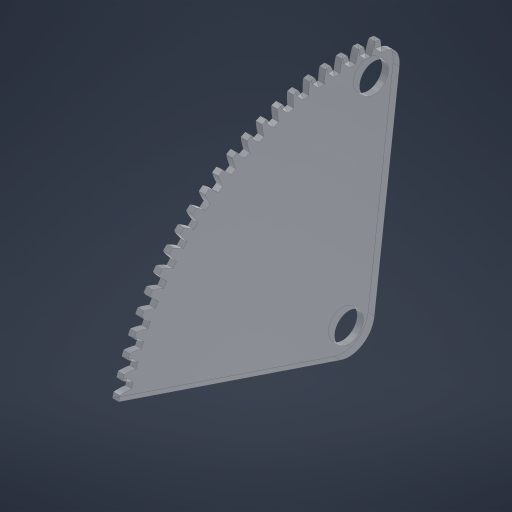
# Autodesk Inventor part: CORL_002_FanPlate
Saved by Autodesk Inventor 2024.2 (Build 282272000, 272)
## iProperties
Created: 2024-08-01
Part Number: CORL_002_FanPlate
Material: Polycarbonate, Clear
Document SubType Name: Modeling
Designer: Bryan
Mass: 353.269 g
Surface Area: 1017.45 cm^2
Volume: 294.391 cm^3
Density: 1.2 g/cm^3
Appearance: Polycarbonate - Clear
Author: Bryan
Autodesk Inventor part; units mm, degrees
ref_plane "YZ Plane" through (0, 0, 0) normal (1, 0, 0) x (0, 1, 0)
ref_plane "XZ Plane" through (0, 0, 0) normal (0, 1, 0) x (-1, 0, 0)
ref_plane "XY Plane" through (0, 0, 0) normal (0, 0, 1) x (1, 0, 0)
sketch "Sketch1" plane through (0, 0, 0) normal (1, 0, 0) x (0, 1, 0)
  circle A0 centre (0, 0) radius 228.6 construction
  circle A1 centre (0, 0) radius 233.68
  circle A2 centre (0, 0) radius 222.25
  line L0 (0, 0) -> (228.6, 0) construction
  line L1 (228.6, 0) -> (214.269, 55.4137) construction
  line L2 (214.269, 55.4137) -> (0, 0) construction
  arc A3 (221.3151, -1.2272) -> (214.269, 55.4137) centre (0, 0) ccw construction
  arc A4 (214.269, 55.4137) -> (209.1377, 72.4107) centre (0, 0) ccw construction
  line L3 (0, 0) -> (222.2162, -3.8788) construction
  line L4 (209.1377, 72.4107) -> (233.6749, 1.542) construction
  spline S0 degree 2 poles (233.6749, 1.542) (228.6917, -0.39) (221.3151, -1.2272) knots 0 0 0 1 1 1
  spline S1 degree 2 poles (233.4787, -9.6962) (228.566, -7.5914) (221.2232, -6.4974) knots 0 0 0 1 1 1
  spline S2 degree 2 poles (232.9981, 17.8386) (228.1618, 15.5636) (220.8616, 14.214) knots 0 0 0 1 1 1
  spline S3 degree 2 poles (233.5864, 6.614) (228.5388, 8.371) (221.1375, 8.9502) knots 0 0 0 1 1 1
  spline S4 degree 2 poles (231.1862, 34.0483) (226.5204, 31.4415) (219.3321, 29.5859) knots 0 0 0 1 1 1
  spline S5 degree 2 poles (232.556, 22.8921) (227.3981, 24.2927) (219.9745, 24.3542) knots 0 0 0 1 1 1
  spline S6 degree 2 poles (228.2479, 50.0921) (223.7753, 47.1662) (216.734, 44.8137) knots 0 0 0 1 1 1
  spline S7 degree 2 poles (230.3926, 39.0586) (225.1496, 40.096) (217.7398, 39.6395) knots 0 0 0 1 1 1
  spline S8 degree 2 poles (224.1977, 65.8918) (219.9401, 62.6611) (213.08, 59.8231) knots 0 0 0 1 1 1
  spline S9 degree 2 poles (227.1068, 55.0348) (221.8042, 55.704) (214.4443, 54.7317) knots 0 0 0 1 1 1
  spline S10 degree 2 poles (219.0552, 81.3706) (215.0333, 77.8507) (208.3879, 74.5411) knots 0 0 0 1 1 1
  spline S11 degree 2 poles (222.7146, 70.7429) (217.3782, 71.0406) (210.104, 69.5573) knots 0 0 0 1 1 1
  spline S12 degree 2 poles (212.8454, 96.4529) (209.0789, 92.661) (202.6806, 88.8959) knots 0 0 0 1 1 1
  spline S13 degree 2 poles (217.2373, 86.1064) (211.8932, 86.0311) (204.7401, 84.0439) knots 0 0 0 1 1 1
  spline S14 degree 2 poles (205.5988, 111.0653) (202.1059, 107.0199) (195.9858, 102.8176) knots 0 0 0 1 1 1
  spline S15 degree 2 poles (210.7016, 101.0504) (205.3758, 100.6024) (198.3788, 98.1211) knots 0 0 0 1 1 1
  spline S16 degree 2 poles (197.3504, 125.1366) (194.1483, 120.8574) (188.3362, 116.2385) knots 0 0 0 1 1 1
  spline S17 degree 2 poles (203.1394, 115.502) (197.8578, 114.6836) (191.051, 111.7203) knots 0 0 0 1 1 1
  spline S18 degree 2 poles (188.1406, 138.5982) (185.2447, 134.1061) (179.769, 129.093) knots 0 0 0 1 1 1
  spline S19 degree 2 poles (194.5876, 129.3909) (189.3759, 128.2061) (182.7923, 124.7752) knots 0 0 0 1 1 1
  spline S20 degree 2 poles (178.0142, 151.3846) (175.4387, 146.7014) (170.326, 141.3186) knots 0 0 0 1 1 1
  spline S21 degree 2 poles (185.0877, 142.6495) (179.9714, 141.104) (173.6432, 137.2222) knots 0 0 0 1 1 1
  spline S22 degree 2 poles (167.0205, 163.4335) (164.778, 158.582) (160.0533, 152.8557) knots 0 0 0 1 1 1
  spline S23 degree 2 poles (174.6861, 155.2131) (169.6901, 153.3145) (163.6481, 149.0007) knots 0 0 0 1 1 1
  spline S24 degree 2 poles (155.2131, 174.6861) (153.3145, 169.6901) (149.0007, 163.6481) knots 0 0 0 1 1 1
  spline S25 degree 2 poles (163.4335, 167.0205) (158.582, 164.778) (152.8557, 160.0533) knots 0 0 0 1 1 1
  spline S26 degree 2 poles (142.6495, 185.0877) (141.104, 179.9714) (137.2222, 173.6432) knots 0 0 0 1 1 1
  spline S27 degree 2 poles (151.3846, 178.0142) (146.7014, 175.4387) (141.3186, 170.326) knots 0 0 0 1 1 1
  spline S28 degree 2 poles (129.3909, 194.5876) (128.2061, 189.3759) (124.7752, 182.7923) knots 0 0 0 1 1 1
  spline S29 degree 2 poles (138.5982, 188.1406) (134.1061, 185.2447) (129.093, 179.769) knots 0 0 0 1 1 1
  spline S30 degree 2 poles (115.502, 203.1394) (114.6836, 197.8578) (111.7203, 191.051) knots 0 0 0 1 1 1
  spline S31 degree 2 poles (125.1366, 197.3504) (120.8574, 194.1483) (116.2385, 188.3362) knots 0 0 0 1 1 1
  spline S32 degree 2 poles (101.0504, 210.7016) (100.6024, 205.3758) (98.1211, 198.3788) knots 0 0 0 1 1 1
  spline S33 degree 2 poles (111.0653, 205.5988) (107.0199, 202.1059) (102.8176, 195.9858) knots 0 0 0 1 1 1
  spline S34 degree 2 poles (86.1064, 217.2373) (86.0311, 211.8932) (84.0439, 204.7401) knots 0 0 0 1 1 1
  spline S35 degree 2 poles (96.4529, 212.8454) (92.661, 209.0789) (88.8959, 202.6806) knots 0 0 0 1 1 1
  spline S36 degree 2 poles (70.7429, 222.7146) (71.0406, 217.3782) (69.5573, 210.104) knots 0 0 0 1 1 1
  spline S37 degree 2 poles (81.3706, 219.0552) (77.8507, 215.0333) (74.5411, 208.3879) knots 0 0 0 1 1 1
  spline S38 degree 2 poles (55.0348, 227.1068) (55.704, 221.8042) (54.7317, 214.4443) knots 0 0 0 1 1 1
  spline S39 degree 2 poles (65.8918, 224.1977) (62.6611, 219.9401) (59.8231, 213.08) knots 0 0 0 1 1 1
  spline S40 degree 2 poles (39.0586, 230.3926) (40.096, 225.1496) (39.6395, 217.7398) knots 0 0 0 1 1 1
  spline S41 degree 2 poles (50.0921, 228.2479) (47.1662, 223.7753) (44.8137, 216.734) knots 0 0 0 1 1 1
  spline S42 degree 2 poles (22.8921, 232.556) (24.2927, 227.3981) (24.3542, 219.9745) knots 0 0 0 1 1 1
  spline S43 degree 2 poles (34.0483, 231.1862) (31.4415, 226.5204) (29.5859, 219.3321) knots 0 0 0 1 1 1
  spline S44 degree 2 poles (6.614, 233.5864) (8.371, 228.5388) (8.9502, 221.1375) knots 0 0 0 1 1 1
  spline S45 degree 2 poles (17.8386, 232.9981) (15.5636, 228.1618) (14.214, 220.8616) knots 0 0 0 1 1 1
  spline S46 degree 2 poles (-9.6962, 233.4787) (-7.5914, 228.566) (-6.4974, 221.2232) knots 0 0 0 1 1 1
  spline S47 degree 2 poles (1.542, 233.6749) (-0.39, 228.6917) (-1.2272, 221.3151) knots 0 0 0 1 1 1
  spline S48 degree 2 poles (-25.9593, 232.2336) (-23.5169, 227.4797) (-21.9133, 220.231) knots 0 0 0 1 1 1
  spline S49 degree 2 poles (-14.7621, 233.2133) (-16.3418, 228.1074) (-16.6623, 220.6904) knots 0 0 0 1 1 1
  spline S50 degree 2 poles (-42.0958, 229.8571) (-39.3278, 225.2851) (-37.2224, 218.166) knots 0 0 0 1 1 1
  spline S51 degree 2 poles (-30.9942, 231.6154) (-32.214, 226.4118) (-32.0163, 218.9905) knots 0 0 0 1 1 1
  spline S52 degree 2 poles (-58.0273, 226.3607) (-54.9471, 221.9929) (-52.3503, 215.038) knots 0 0 0 1 1 1
  spline S53 degree 2 poles (-47.0754, 228.8892) (-47.9292, 223.6132) (-47.2144, 216.2237) knots 0 0 0 1 1 1
  spline S54 degree 2 poles (-73.6761, 221.7615) (-70.2987, 217.6193) (-67.223, 210.8624) knots 0 0 0 1 1 1
  spline S55 degree 2 poles (-62.9272, 225.0478) (-63.4109, 219.7251) (-62.1824, 212.4035) knots 0 0 0 1 1 1
  spline S56 degree 2 poles (-88.9659, 216.0819) (-85.3078, 212.1854) (-81.7683, 205.6595) knots 0 0 0 1 1 1
  spline S57 degree 2 poles (-78.4725, 220.11) (-78.5837, 214.7665) (-76.8474, 207.5485) knots 0 0 0 1 1 1
  spline S58 degree 2 poles (-103.8223, 209.3496) (-99.9013, 205.7177) (-95.9152, 199.4547) knots 0 0 0 1 1 1
  spline S59 degree 2 poles (-93.6354, 214.0999) (-93.3736, 208.7616) (-91.1381, 201.6823) knots 0 0 0 1 1 1
  spline S60 degree 2 poles (-118.1729, 201.5974) (-114.0081, 198.2478) (-109.5948, 192.2781) knots 0 0 0 1 1 1
  spline S61 degree 2 poles (-108.3422, 207.0466) (-107.7086, 201.7397) (-104.9847, 194.8336) knots 0 0 0 1 1 1
  spline S62 degree 2 poles (-131.9478, 192.863) (-127.5594, 189.8121) (-122.7405, 184.1648) knots 0 0 0 1 1 1
  spline S63 degree 2 poles (-122.5211, 198.9847) (-121.5189, 193.7349) (-118.3199, 187.0356) knots 0 0 0 1 1 1
  spline S64 degree 2 poles (-145.0798, 183.189) (-140.4893, 180.4517) (-135.2882, 175.1542) knots 0 0 0 1 1 1
  spline S65 degree 2 poles (-136.1031, 189.9534) (-134.7372, 184.7862) (-131.0786, 178.3264) knots 0 0 0 1 1 1
  spline S66 degree 2 poles (-157.505, 172.6225) (-152.7348, 170.212) (-147.1768, 165.2903) knots 0 0 0 1 1 1
  spline S67 degree 2 poles (-149.0221, 179.9966) (-147.299, 174.9373) (-143.1987, 168.7484) knots 0 0 0 1 1 1
  spline S68 degree 2 poles (-169.1629, 161.215) (-164.2361, 159.1432) (-158.3483, 154.6212) knots 0 0 0 1 1 1
  spline S69 degree 2 poles (-161.215, 169.1629) (-159.1432, 164.2361) (-154.6212, 158.3483) knots 0 0 0 1 1 1
  spline S70 degree 2 poles (-179.9966, 149.0221) (-174.9373, 147.299) (-168.7484, 143.1987) knots 0 0 0 1 1 1
  spline S71 degree 2 poles (-172.6225, 157.505) (-170.212, 152.7348) (-165.2903, 147.1768) knots 0 0 0 1 1 1
  spline S72 degree 2 poles (-189.9534, 136.1031) (-184.7862, 134.7372) (-178.3264, 131.0786) knots 0 0 0 1 1 1
  spline S73 degree 2 poles (-183.189, 145.0798) (-180.4517, 140.4893) (-175.1542, 135.2882) knots 0 0 0 1 1 1
  spline S74 degree 2 poles (-198.9847, 122.5211) (-193.7349, 121.5189) (-187.0356, 118.3199) knots 0 0 0 1 1 1
  spline S75 degree 2 poles (-192.863, 131.9478) (-189.8121, 127.5594) (-184.1648, 122.7405) knots 0 0 0 1 1 1
  spline S76 degree 2 poles (-207.0466, 108.3422) (-201.7397, 107.7086) (-194.8336, 104.9847) knots 0 0 0 1 1 1
  spline S77 degree 2 poles (-201.5974, 118.1729) (-198.2478, 114.0081) (-192.2781, 109.5948) knots 0 0 0 1 1 1
  spline S78 degree 2 poles (-214.0999, 93.6354) (-208.7616, 93.3736) (-201.6823, 91.1381) knots 0 0 0 1 1 1
  spline S79 degree 2 poles (-209.3496, 103.8223) (-205.7177, 99.9013) (-199.4547, 95.9152) knots 0 0 0 1 1 1
  spline S80 degree 2 poles (-220.11, 78.4725) (-214.7665, 78.5837) (-207.5485, 76.8474) knots 0 0 0 1 1 1
  spline S81 degree 2 poles (-216.0819, 88.9659) (-212.1854, 85.3078) (-205.6595, 81.7683) knots 0 0 0 1 1 1
  spline S82 degree 2 poles (-225.0478, 62.9272) (-219.7251, 63.4109) (-212.4035, 62.1824) knots 0 0 0 1 1 1
  spline S83 degree 2 poles (-221.7615, 73.6761) (-217.6193, 70.2987) (-210.8624, 67.223) knots 0 0 0 1 1 1
  spline S84 degree 2 poles (-228.8892, 47.0754) (-223.6132, 47.9292) (-216.2237, 47.2144) knots 0 0 0 1 1 1
  spline S85 degree 2 poles (-226.3607, 58.0273) (-221.9929, 54.9471) (-215.038, 52.3503) knots 0 0 0 1 1 1
  spline S86 degree 2 poles (-231.6154, 30.9942) (-226.4118, 32.214) (-218.9905, 32.0163) knots 0 0 0 1 1 1
  spline S87 degree 2 poles (-229.8571, 42.0958) (-225.2851, 39.3278) (-218.166, 37.2224) knots 0 0 0 1 1 1
  spline S88 degree 2 poles (-233.2133, 14.7621) (-228.1074, 16.3418) (-220.6904, 16.6623) knots 0 0 0 1 1 1
  spline S89 degree 2 poles (-232.2336, 25.9593) (-227.4797, 23.5169) (-220.231, 21.9133) knots 0 0 0 1 1 1
  spline S90 degree 2 poles (-233.6749, -1.542) (-228.6917, 0.39) (-221.3151, 1.2272) knots 0 0 0 1 1 1
  spline S91 degree 2 poles (-233.4787, 9.6962) (-228.566, 7.5914) (-221.2232, 6.4974) knots 0 0 0 1 1 1
  spline S92 degree 2 poles (-232.9981, -17.8386) (-228.1618, -15.5636) (-220.8616, -14.214) knots 0 0 0 1 1 1
  spline S93 degree 2 poles (-233.5864, -6.614) (-228.5388, -8.371) (-221.1375, -8.9502) knots 0 0 0 1 1 1
  spline S94 degree 2 poles (-231.1862, -34.0483) (-226.5204, -31.4415) (-219.3321, -29.5859) knots 0 0 0 1 1 1
  spline S95 degree 2 poles (-232.556, -22.8921) (-227.3981, -24.2927) (-219.9745, -24.3542) knots 0 0 0 1 1 1
  spline S96 degree 2 poles (-228.2479, -50.0921) (-223.7753, -47.1662) (-216.734, -44.8137) knots 0 0 0 1 1 1
  spline S97 degree 2 poles (-230.3926, -39.0586) (-225.1496, -40.096) (-217.7398, -39.6395) knots 0 0 0 1 1 1
  spline S98 degree 2 poles (-224.1977, -65.8918) (-219.9401, -62.6611) (-213.08, -59.8231) knots 0 0 0 1 1 1
  spline S99 degree 2 poles (-227.1068, -55.0348) (-221.8042, -55.704) (-214.4443, -54.7317) knots 0 0 0 1 1 1
  spline S100 degree 2 poles (-219.0552, -81.3706) (-215.0333, -77.8507) (-208.3879, -74.5411) knots 0 0 0 1 1 1
  spline S101 degree 2 poles (-222.7146, -70.7429) (-217.3782, -71.0406) (-210.104, -69.5573) knots 0 0 0 1 1 1
  spline S102 degree 2 poles (-212.8454, -96.4529) (-209.0789, -92.661) (-202.6806, -88.8959) knots 0 0 0 1 1 1
  spline S103 degree 2 poles (-217.2373, -86.1064) (-211.8932, -86.0311) (-204.7401, -84.0439) knots 0 0 0 1 1 1
  spline S104 degree 2 poles (-205.5988, -111.0653) (-202.1059, -107.0199) (-195.9858, -102.8176) knots 0 0 0 1 1 1
  spline S105 degree 2 poles (-210.7016, -101.0504) (-205.3758, -100.6024) (-198.3788, -98.1211) knots 0 0 0 1 1 1
  spline S106 degree 2 poles (-197.3504, -125.1366) (-194.1483, -120.8574) (-188.3362, -116.2385) knots 0 0 0 1 1 1
  spline S107 degree 2 poles (-203.1394, -115.502) (-197.8578, -114.6836) (-191.051, -111.7203) knots 0 0 0 1 1 1
  spline S108 degree 2 poles (-188.1406, -138.5982) (-185.2447, -134.1061) (-179.769, -129.093) knots 0 0 0 1 1 1
  spline S109 degree 2 poles (-194.5876, -129.3909) (-189.3759, -128.2061) (-182.7923, -124.7752) knots 0 0 0 1 1 1
  spline S110 degree 2 poles (-178.0142, -151.3846) (-175.4387, -146.7014) (-170.326, -141.3186) knots 0 0 0 1 1 1
  spline S111 degree 2 poles (-185.0877, -142.6495) (-179.9714, -141.104) (-173.6432, -137.2222) knots 0 0 0 1 1 1
  spline S112 degree 2 poles (-167.0205, -163.4335) (-164.778, -158.582) (-160.0533, -152.8557) knots 0 0 0 1 1 1
  spline S113 degree 2 poles (-174.6861, -155.2131) (-169.6901, -153.3145) (-163.6481, -149.0007) knots 0 0 0 1 1 1
  spline S114 degree 2 poles (-155.2131, -174.6861) (-153.3145, -169.6901) (-149.0007, -163.6481) knots 0 0 0 1 1 1
  spline S115 degree 2 poles (-163.4335, -167.0205) (-158.582, -164.778) (-152.8557, -160.0533) knots 0 0 0 1 1 1
  spline S116 degree 2 poles (-142.6495, -185.0877) (-141.104, -179.9714) (-137.2222, -173.6432) knots 0 0 0 1 1 1
  spline S117 degree 2 poles (-151.3846, -178.0142) (-146.7014, -175.4387) (-141.3186, -170.326) knots 0 0 0 1 1 1
  spline S118 degree 2 poles (-129.3909, -194.5876) (-128.2061, -189.3759) (-124.7752, -182.7923) knots 0 0 0 1 1 1
  spline S119 degree 2 poles (-138.5982, -188.1406) (-134.1061, -185.2447) (-129.093, -179.769) knots 0 0 0 1 1 1
  spline S120 degree 2 poles (-115.502, -203.1394) (-114.6836, -197.8578) (-111.7203, -191.051) knots 0 0 0 1 1 1
  spline S121 degree 2 poles (-125.1366, -197.3504) (-120.8574, -194.1483) (-116.2385, -188.3362) knots 0 0 0 1 1 1
  spline S122 degree 2 poles (-101.0504, -210.7016) (-100.6024, -205.3758) (-98.1211, -198.3788) knots 0 0 0 1 1 1
  spline S123 degree 2 poles (-111.0653, -205.5988) (-107.0199, -202.1059) (-102.8176, -195.9858) knots 0 0 0 1 1 1
  spline S124 degree 2 poles (-86.1064, -217.2373) (-86.0311, -211.8932) (-84.0439, -204.7401) knots 0 0 0 1 1 1
  spline S125 degree 2 poles (-96.4529, -212.8454) (-92.661, -209.0789) (-88.8959, -202.6806) knots 0 0 0 1 1 1
  spline S126 degree 2 poles (-70.7429, -222.7146) (-71.0406, -217.3782) (-69.5573, -210.104) knots 0 0 0 1 1 1
  spline S127 degree 2 poles (-81.3706, -219.0552) (-77.8507, -215.0333) (-74.5411, -208.3879) knots 0 0 0 1 1 1
  spline S128 degree 2 poles (-55.0348, -227.1068) (-55.704, -221.8042) (-54.7317, -214.4443) knots 0 0 0 1 1 1
  spline S129 degree 2 poles (-65.8918, -224.1977) (-62.6611, -219.9401) (-59.8231, -213.08) knots 0 0 0 1 1 1
  spline S130 degree 2 poles (-39.0586, -230.3926) (-40.096, -225.1496) (-39.6395, -217.7398) knots 0 0 0 1 1 1
  spline S131 degree 2 poles (-50.0921, -228.2479) (-47.1662, -223.7753) (-44.8137, -216.734) knots 0 0 0 1 1 1
  spline S132 degree 2 poles (-22.8921, -232.556) (-24.2927, -227.3981) (-24.3542, -219.9745) knots 0 0 0 1 1 1
  spline S133 degree 2 poles (-34.0483, -231.1862) (-31.4415, -226.5204) (-29.5859, -219.3321) knots 0 0 0 1 1 1
  spline S134 degree 2 poles (-6.614, -233.5864) (-8.371, -228.5388) (-8.9502, -221.1375) knots 0 0 0 1 1 1
  spline S135 degree 2 poles (-17.8386, -232.9981) (-15.5636, -228.1618) (-14.214, -220.8616) knots 0 0 0 1 1 1
  spline S136 degree 2 poles (9.6962, -233.4787) (7.5914, -228.566) (6.4974, -221.2232) knots 0 0 0 1 1 1
  spline S137 degree 2 poles (-1.542, -233.6749) (0.39, -228.6917) (1.2272, -221.3151) knots 0 0 0 1 1 1
  spline S138 degree 2 poles (25.9593, -232.2336) (23.5169, -227.4797) (21.9133, -220.231) knots 0 0 0 1 1 1
  spline S139 degree 2 poles (14.7621, -233.2133) (16.3418, -228.1074) (16.6623, -220.6904) knots 0 0 0 1 1 1
  spline S140 degree 2 poles (42.0958, -229.8571) (39.3278, -225.2851) (37.2224, -218.166) knots 0 0 0 1 1 1
  spline S141 degree 2 poles (30.9942, -231.6154) (32.214, -226.4118) (32.0163, -218.9905) knots 0 0 0 1 1 1
  spline S142 degree 2 poles (58.0273, -226.3607) (54.9471, -221.9929) (52.3503, -215.038) knots 0 0 0 1 1 1
  spline S143 degree 2 poles (47.0754, -228.8892) (47.9292, -223.6132) (47.2144, -216.2237) knots 0 0 0 1 1 1
  spline S144 degree 2 poles (73.6761, -221.7615) (70.2987, -217.6193) (67.223, -210.8624) knots 0 0 0 1 1 1
  spline S145 degree 2 poles (62.9272, -225.0478) (63.4109, -219.7251) (62.1824, -212.4035) knots 0 0 0 1 1 1
  spline S146 degree 2 poles (88.9659, -216.0819) (85.3078, -212.1854) (81.7683, -205.6595) knots 0 0 0 1 1 1
  spline S147 degree 2 poles (78.4725, -220.11) (78.5837, -214.7665) (76.8474, -207.5485) knots 0 0 0 1 1 1
  spline S148 degree 2 poles (103.8223, -209.3496) (99.9013, -205.7177) (95.9152, -199.4547) knots 0 0 0 1 1 1
  spline S149 degree 2 poles (93.6354, -214.0999) (93.3736, -208.7616) (91.1381, -201.6823) knots 0 0 0 1 1 1
  spline S150 degree 2 poles (118.1729, -201.5974) (114.0081, -198.2478) (109.5948, -192.2781) knots 0 0 0 1 1 1
  spline S151 degree 2 poles (108.3422, -207.0466) (107.7086, -201.7397) (104.9847, -194.8336) knots 0 0 0 1 1 1
  spline S152 degree 2 poles (131.9478, -192.863) (127.5594, -189.8121) (122.7405, -184.1648) knots 0 0 0 1 1 1
  spline S153 degree 2 poles (122.5211, -198.9847) (121.5189, -193.7349) (118.3199, -187.0356) knots 0 0 0 1 1 1
  spline S154 degree 2 poles (145.0798, -183.189) (140.4893, -180.4517) (135.2882, -175.1542) knots 0 0 0 1 1 1
  spline S155 degree 2 poles (136.1031, -189.9534) (134.7372, -184.7862) (131.0786, -178.3264) knots 0 0 0 1 1 1
  spline S156 degree 2 poles (157.505, -172.6225) (152.7348, -170.212) (147.1768, -165.2903) knots 0 0 0 1 1 1
  spline S157 degree 2 poles (149.0221, -179.9966) (147.299, -174.9373) (143.1987, -168.7484) knots 0 0 0 1 1 1
  spline S158 degree 2 poles (169.1629, -161.215) (164.2361, -159.1432) (158.3483, -154.6212) knots 0 0 0 1 1 1
  spline S159 degree 2 poles (161.215, -169.1629) (159.1432, -164.2361) (154.6212, -158.3483) knots 0 0 0 1 1 1
  spline S160 degree 2 poles (179.9966, -149.0221) (174.9373, -147.299) (168.7484, -143.1987) knots 0 0 0 1 1 1
  spline S161 degree 2 poles (172.6225, -157.505) (170.212, -152.7348) (165.2903, -147.1768) knots 0 0 0 1 1 1
  spline S162 degree 2 poles (189.9534, -136.1031) (184.7862, -134.7372) (178.3264, -131.0786) knots 0 0 0 1 1 1
  spline S163 degree 2 poles (183.189, -145.0798) (180.4517, -140.4893) (175.1542, -135.2882) knots 0 0 0 1 1 1
  spline S164 degree 2 poles (198.9847, -122.5211) (193.7349, -121.5189) (187.0356, -118.3199) knots 0 0 0 1 1 1
  spline S165 degree 2 poles (192.863, -131.9478) (189.8121, -127.5594) (184.1648, -122.7405) knots 0 0 0 1 1 1
  spline S166 degree 2 poles (207.0466, -108.3422) (201.7397, -107.7086) (194.8336, -104.9847) knots 0 0 0 1 1 1
  spline S167 degree 2 poles (201.5974, -118.1729) (198.2478, -114.0081) (192.2781, -109.5948) knots 0 0 0 1 1 1
  spline S168 degree 2 poles (214.0999, -93.6354) (208.7616, -93.3736) (201.6823, -91.1381) knots 0 0 0 1 1 1
  spline S169 degree 2 poles (209.3496, -103.8223) (205.7177, -99.9013) (199.4547, -95.9152) knots 0 0 0 1 1 1
  spline S170 degree 2 poles (220.11, -78.4725) (214.7665, -78.5837) (207.5485, -76.8474) knots 0 0 0 1 1 1
  spline S171 degree 2 poles (216.0819, -88.9659) (212.1854, -85.3078) (205.6595, -81.7683) knots 0 0 0 1 1 1
  spline S172 degree 2 poles (225.0478, -62.9272) (219.7251, -63.4109) (212.4035, -62.1824) knots 0 0 0 1 1 1
  spline S173 degree 2 poles (221.7615, -73.6761) (217.6193, -70.2987) (210.8624, -67.223) knots 0 0 0 1 1 1
  spline S174 degree 2 poles (228.8892, -47.0754) (223.6132, -47.9292) (216.2237, -47.2144) knots 0 0 0 1 1 1
  spline S175 degree 2 poles (226.3607, -58.0273) (221.9929, -54.9471) (215.038, -52.3503) knots 0 0 0 1 1 1
  spline S176 degree 2 poles (231.6154, -30.9942) (226.4118, -32.214) (218.9905, -32.0163) knots 0 0 0 1 1 1
  spline S177 degree 2 poles (229.8571, -42.0958) (225.2851, -39.3278) (218.166, -37.2224) knots 0 0 0 1 1 1
  spline S178 degree 2 poles (233.2133, -14.7621) (228.1074, -16.3418) (220.6904, -16.6623) knots 0 0 0 1 1 1
  spline S179 degree 2 poles (232.2336, -25.9593) (227.4797, -23.5169) (220.231, -21.9133) knots 0 0 0 1 1 1
  point P0 (228.4607, -7.978)
  point P1 (228.0431, 15.9463)
  point P2 (228.4607, 7.978)
  point P3 (226.3753, 31.815)
  point P4 (227.3477, 23.8952)
  point P5 (223.6045, 47.5286)
  point P6 (225.1271, 39.696)
  point P7 (219.7444, 63.0107)
  point P8 (221.8096, 55.3033)
  point P9 (214.8137, 78.1858)
  point P10 (217.4115, 70.6413)
  point P11 (208.8365, 92.98)
  point P12 (211.9542, 85.6351)
  point P13 (201.8418, 107.3212)
  point P14 (205.4643, 100.2116)
  point P15 (193.8638, 121.1395)
  point P16 (197.9734, 114.3)
  point P17 (184.9413, 134.3677)
  point P18 (189.518, 127.8315)
  point P19 (175.1178, 146.9412)
  point P20 (180.1393, 140.7402)
  point P21 (164.4411, 158.7989)
  point P22 (169.8829, 152.9633)
  point P23 (152.9633, 169.8829)
  point P24 (158.7989, 164.4411)
  point P25 (140.7402, 180.1393)
  point P26 (146.9412, 175.1178)
  point P27 (127.8315, 189.518)
  point P28 (134.3677, 184.9413)
  point P29 (114.3, 197.9734)
  point P30 (121.1395, 193.8638)
  point P31 (100.2116, 205.4643)
  point P32 (107.3212, 201.8418)
  point P33 (85.6351, 211.9542)
  point P34 (92.98, 208.8365)
  point P35 (70.6413, 217.4115)
  point P36 (78.1858, 214.8137)
  point P37 (55.3033, 221.8096)
  point P38 (63.0107, 219.7444)
  point P39 (39.696, 225.1271)
  point P40 (47.5286, 223.6045)
  point P41 (23.8952, 227.3477)
  point P42 (31.815, 226.3753)
  point P43 (7.978, 228.4607)
  point P44 (15.9463, 228.0431)
  point P45 (-7.978, 228.4607)
  point P46 (0, 228.6)
  point P47 (-23.8952, 227.3477)
  point P48 (-15.9463, 228.0431)
  point P49 (-39.696, 225.1271)
  point P50 (-31.815, 226.3753)
  point P51 (-55.3033, 221.8096)
  point P52 (-47.5286, 223.6045)
  point P53 (-70.6413, 217.4115)
  point P54 (-63.0107, 219.7444)
  point P55 (-85.6351, 211.9542)
  point P56 (-78.1858, 214.8137)
  point P57 (-100.2116, 205.4643)
  point P58 (-92.98, 208.8365)
  point P59 (-114.3, 197.9734)
  point P60 (-107.3212, 201.8418)
  point P61 (-127.8315, 189.518)
  point P62 (-121.1395, 193.8638)
  point P63 (-140.7402, 180.1393)
  point P64 (-134.3677, 184.9413)
  point P65 (-152.9633, 169.8829)
  point P66 (-146.9412, 175.1178)
  point P67 (-164.4411, 158.7989)
  point P68 (-158.7989, 164.4411)
  point P69 (-175.1178, 146.9412)
  point P70 (-169.8829, 152.9633)
  point P71 (-184.9413, 134.3677)
  point P72 (-180.1393, 140.7402)
  point P73 (-193.8638, 121.1395)
  point P74 (-189.518, 127.8315)
  point P75 (-201.8418, 107.3212)
  point P76 (-197.9734, 114.3)
  point P77 (-208.8365, 92.98)
  point P78 (-205.4643, 100.2116)
  point P79 (-214.8137, 78.1858)
  point P80 (-211.9542, 85.6351)
  point P81 (-219.7444, 63.0107)
  point P82 (-217.4115, 70.6413)
  point P83 (-223.6045, 47.5286)
  point P84 (-221.8096, 55.3033)
  point P85 (-226.3753, 31.815)
  point P86 (-225.1271, 39.696)
  point P87 (-228.0431, 15.9463)
  point P88 (-227.3477, 23.8952)
  point P89 (-228.6, 0)
  point P90 (-228.4607, 7.978)
  point P91 (-228.0431, -15.9463)
  point P92 (-228.4607, -7.978)
  point P93 (-226.3753, -31.815)
  point P94 (-227.3477, -23.8952)
  point P95 (-223.6045, -47.5286)
  point P96 (-225.1271, -39.696)
  point P97 (-219.7444, -63.0107)
  point P98 (-221.8096, -55.3033)
  point P99 (-214.8137, -78.1858)
  point P100 (-217.4115, -70.6413)
  point P101 (-208.8365, -92.98)
  point P102 (-211.9542, -85.6351)
  point P103 (-201.8418, -107.3212)
  point P104 (-205.4643, -100.2116)
  point P105 (-193.8638, -121.1395)
  point P106 (-197.9734, -114.3)
  point P107 (-184.9413, -134.3677)
  point P108 (-189.518, -127.8315)
  point P109 (-175.1178, -146.9412)
  point P110 (-180.1393, -140.7402)
  point P111 (-164.4411, -158.7989)
  point P112 (-169.8829, -152.9633)
  point P113 (-152.9633, -169.8829)
  point P114 (-158.7989, -164.4411)
  point P115 (-140.7402, -180.1393)
  point P116 (-146.9412, -175.1178)
  point P117 (-127.8315, -189.518)
  point P118 (-134.3677, -184.9413)
  point P119 (-114.3, -197.9734)
  point P120 (-121.1395, -193.8638)
  point P121 (-100.2116, -205.4643)
  point P122 (-107.3212, -201.8418)
  point P123 (-85.6351, -211.9542)
  point P124 (-92.98, -208.8365)
  point P125 (-70.6413, -217.4115)
  point P126 (-78.1858, -214.8137)
  point P127 (-55.3033, -221.8096)
  point P128 (-63.0107, -219.7444)
  point P129 (-39.696, -225.1271)
  point P130 (-47.5286, -223.6045)
  point P131 (-23.8952, -227.3477)
  point P132 (-31.815, -226.3753)
  point P133 (-7.978, -228.4607)
  point P134 (-15.9463, -228.0431)
  point P135 (7.978, -228.4607)
  point P136 (0, -228.6)
  point P137 (23.8952, -227.3477)
  point P138 (15.9463, -228.0431)
  point P139 (39.696, -225.1271)
  point P140 (31.815, -226.3753)
  point P141 (55.3033, -221.8096)
  point P142 (47.5286, -223.6045)
  point P143 (70.6413, -217.4115)
  point P144 (63.0107, -219.7444)
  point P145 (85.6351, -211.9542)
  point P146 (78.1858, -214.8137)
  point P147 (100.2116, -205.4643)
  point P148 (92.98, -208.8365)
  point P149 (114.3, -197.9734)
  point P150 (107.3212, -201.8418)
  point P151 (127.8315, -189.518)
  point P152 (121.1395, -193.8638)
  point P153 (140.7402, -180.1393)
  point P154 (134.3677, -184.9413)
  point P155 (152.9633, -169.8829)
  point P156 (146.9412, -175.1178)
  point P157 (164.4411, -158.7989)
  point P158 (158.7989, -164.4411)
  point P159 (175.1178, -146.9412)
  point P160 (169.8829, -152.9633)
  point P161 (184.9413, -134.3677)
  point P162 (180.1393, -140.7402)
  point P163 (193.8638, -121.1395)
  point P164 (189.518, -127.8315)
  point P165 (201.8418, -107.3212)
  point P166 (197.9734, -114.3)
  point P167 (208.8365, -92.98)
  point P168 (205.4643, -100.2116)
  point P169 (214.8137, -78.1858)
  point P170 (211.9542, -85.6351)
  point P171 (219.7444, -63.0107)
  point P172 (217.4115, -70.6413)
  point P173 (223.6045, -47.5286)
  point P174 (221.8096, -55.3033)
  point P175 (226.3753, -31.815)
  point P176 (225.1271, -39.696)
  point P177 (228.0431, -15.9463)
  point P178 (227.3477, -23.8952)
  point P179 (-110.1573, 193.0296)
  point P180 (-118.1729, 201.5974)
  point P181 (229.8571, -42.0958)
  point P182 (219.0645, -37.4939)
  point P183 (219.929, -32.0358)
  point P184 (231.6154, -30.9942)
  point P185 (232.2336, -25.9593)
  point P186 (221.1463, -22.1214)
  point P187 (221.628, -16.6163)
  point P188 (233.2133, -14.7621)
  point P189 (233.4787, -9.6962)
  point P190 (222.1508, -6.6412)
  point P191 (222.2472, -1.1158)
  point P192 (233.5864, 6.614)
  point P193 (222.0729, 8.8715)
  point P194 (221.7837, 14.3901)
  point P195 (232.9981, 17.8386)
  point P196 (232.556, 22.8921)
  point P197 (220.9131, 24.3409)
  point P198 (220.2396, 29.8259)
  point P199 (231.1862, 34.0483)
  dimension "d18" = 457.2
  dimension "d19" = 467.36
  dimension "d20" = 444.5
  dimension "d21" = 14.5
  dimension "d22" = 57.2369
  dimension "d23" = 57.2369
  dimension "d26" = 1
  dimension "d61" = 74.9963
  dimension "d62" = 17.7594
  dimension "d65" = 360
  constraints: 10 end point, 4 point on circle, 3 coincident, 3 symmetric about line, 2 centre point, 2 tangent, 1 horizontal, 1 horizontal alignment, 1 perpendicular, 1271 other
  measures "d21" angle of L0 L2
  measures "d22" distance of L0.end L1.end
  measures "d26" angle of L3 L0
  measures "d61" distance of L4.start L4.end
extrude "Extrusion2" add sketch "Sketch1" along normal blind 6.35 contours S0 A2 S3 A1 | A1 S178 A2 S1 | A2 | S2 A2 S5 A1 | A1 S176 A2 S179 | S4 A2 S7 A1 | A1 S174 A2 S177 | A1 S175 A2 S174 | S6 A2 S9 A1 | A1 S172 A2 S175 | A1 S173 A2 S172 | S8 A2 S11 A1 | A1 S170 A2 S173 | A1 S171 A2 S170 | S10 A2 S13 A1 | A1 S168 A2 S171 | A1 S169 A2 S168 | S12 A2 S15 A1 | A1 S166 A2 S169 | A1 S167 A2 S166 | S14 A2 S17 A1 | A1 S164 A2 S167 | A1 S165 A2 S164 | S16 A2 S19 A1 | A1 S162 A2 S165 | A1 S163 A2 S162 | S18 A2 S21 A1 | A1 S160 A2 S163 | A1 S161 A2 S160 | S20 A2 S23 A1 | A1 S158 A2 S161 | A1 S159 A2 S158 | S22 A2 S25 A1 | A1 S156 A2 S159 | A1 S157 A2 S156 | S24 A2 S27 A1 | A1 S154 A2 S157 | A1 S155 A2 S154 | S26 A2 S29 A1 | A1 S152 A2 S155 | A1 S153 A2 S152 | S28 A2 S31 A1 | A1 S150 A2 S153 | A1 S151 A2 S150 | S30 A2 S33 A1 | A1 S148 A2 S151 | A1 S149 A2 S148 | S32 A2 S35 A1 | A1 S146 A2 S149 | A1 S147 A2 S146 | S34 A2 S37 A1 | A1 S144 A2 S147 | A1 S145 A2 S144 | S36 A2 S39 A1 | A1 S142 A2 S145 | A1 S143 A2 S142 | S38 A2 S41 A1 | A1 S140 A2 S143 | A1 S141 A2 S140 | S40 A2 S43 A1 | A1 S138 A2 S141 | A1 S139 A2 S138 | S42 A2 S45 A1 | A1 S136 A2 S139 | A1 S137 A2 S136 | S44 A2 S47 A1 | A1 S134 A2 S137 | A1 S135 A2 S134 | S46 A2 S49 A1 | A1 S132 A2 S135 | A1 S133 A2 S132 | S48 A2 S51 A1 | A1 S130 A2 S133 | A1 S131 A2 S130 | S50 A2 S53 A1 | A1 S128 A2 S131 | A1 S129 A2 S128 | S52 A2 S55 A1 | A1 S126 A2 S129 | A1 S127 A2 S126 | S54 A2 S57 A1 | A1 S124 A2 S127 | A1 S125 A2 S124 | S56 A2 S59 A1 | A1 S122 A2 S125 | A1 S123 A2 S122 | S58 A2 S61 A1 | A1 S120 A2 S123 | A1 S121 A2 S120 | S60 A2 S63 A1 | A1 S118 A2 S121 | S63 A2 S62 A1 | A1 S119 A2 S118 | S62 A2 S65 A1 | A1 S116 A2 S119 | S65 A2 S64 A1 | A1 S117 A2 S116 | S64 A2 S67 A1 | A1 S114 A2 S117 | S67 A2 S66 A1 | A1 S115 A2 S114 | S66 A2 S69 A1 | A1 S112 A2 S115 | S69 A2 S68 A1 | A1 S113 A2 S112 | S68 A2 S71 A1 | A1 S110 A2 S113 | S71 A2 S70 A1 | A1 S111 A2 S110 | S70 A2 S73 A1 | A1 S108 A2 S111 | S73 A2 S72 A1 | A1 S109 A2 S108 | S72 A2 S75 A1 | A1 S106 A2 S109 | S75 A2 S74 A1 | A1 S107 A2 S106 | S74 A2 S77 A1 | A1 S104 A2 S107 | S77 A2 S76 A1 | A1 S105 A2 S104 | S76 A2 S79 A1 | A1 S102 A2 S105 | S79 A2 S78 A1 | A1 S103 A2 S102 | S78 A2 S81 A1 | A1 S100 A2 S103 | S81 A2 S80 A1 | A1 S101 A2 S100 | S80 A2 S83 A1 | A1 S98 A2 S101 | S83 A2 S82 A1 | A1 S99 A2 S98 | S82 A2 S85 A1 | A1 S96 A2 S99 | S85 A2 S84 A1 | A1 S97 A2 S96 | S84 A2 S87 A1 | A1 S94 A2 S97 | S87 A2 S86 A1 | A1 S95 A2 S94 | S86 A2 S89 A1 | A1 S92 A2 S95 | S89 A2 S88 A1 | A1 S93 A2 S92 | S88 A2 S91 A1 | A1 S90 A2 S93 | S91 A2 S90 A1
sketch "Sketch11" plane through (6.35, 0, 0) normal (1, 0, 0) x (0, 0, -1)
  circle A0 centre (0, 0) radius 14.2875
  line L0 (0, 0) -> (28.4784, 231.9382)
  circle A1 centre (24.7639, 201.6854) radius 50.8
  circle A2 centre (24.7639, 201.6854) radius 14.2875
  line L1 (0, 0) -> (-222.3361, 53.147)
  line L2 (24.7639, 201.6854) -> (27.8593, 226.8961)
  arc A3 (27.8593, 226.8961) -> (-222.3361, 53.147) centre (0, 0) ccw
  circle A4 centre (0, 0) radius 233.68
  line L3 (-222.3361, 53.147) -> (-227.2769, 54.328)
  circle A5 centre (24.7639, 201.6854) radius 25.4
  arc A6 (6.6412, 222.1508) -> (1.1158, 222.2472) centre (0, 0) ccw projected
  line L4 (49.9745, 198.5899) -> (25.2107, -3.0955)
  circle A7 centre (0, 0) radius 25.4
  arc A8 (30.9942, 231.6154) -> (25.9593, 232.2336) centre (0, 0) ccw projected
  line L5 (-228.2479, 50.0921) -> (-8.1092, -24.0707)
  spline S0 degree 2 poles (32.0358, 219.929) (32.1361, 226.744) (30.9942, 231.6154) knots 0 0 0 1 1 1 projected
  point P0 (14.7621, 233.2133)
  point P1 (-24.704, 5.9052)
  point P2 (14.7621, 233.2133)
  point P3 (27.8593, 226.8961)
  point P4 (27.8593, 226.8961)
  point P5 (3.0955, 25.2107)
  point P6 (21.6684, 176.4747)
  point P7 (-13.896, 3.3217)
  point P8 (1.7412, 14.181)
  point P9 (31.8411, 226.0795)
  dimension "d79" = 50.8
  dimension "d67" = 28.575
  dimension "d68" = 101.6
  dimension "d69" = 28.575
  dimension "d70" = 203.2
  dimension "d71" = 228.6
  dimension "d75" = 83.556
  dimension "d76" = 25.4
  dimension "d77" = 333.375
  dimension "d78" = 467.36
  dimension "d80" = 50.8
  constraints: 12 end point, 6 centre point, 6 point on circle, 5 coincident, 2 point on line, 2 tangent, 1 collinear, 7 other
  measures "d67" diameter of A0
  measures "d68" diameter of A1
  measures "d69" diameter of A2
  measures "d70" distance of point (0, 0) A1.centre
  measures "d71" distance of L0.start L1.end
  measures "d75" angle of L1 L0
  measures "d76" distance of L2.start L2.end
  measures "d78" diameter of A4
  measures "d80" diameter of A7
extrude "Extrusion12" cut sketch "Sketch11" against normal blind 6.35 contours A0 L1 L0 | L0 L1 A0 | A7 L4 A1 A4 L5 | L4 A5 S0 A4 A1 | A2 L0 | L0 A2
sketch "Sketch12" plane through (6.35, 0, 0) normal (1, 0, 0) x (0, 0, -1)
  circle A0 centre (24.7639, 201.6854) radius 14.2875 projected
  arc A1 (30.9942, 231.6154) -> (25.9593, 232.2336) centre (0, 0) ccw projected
  arc A2 (22.1214, 221.1463) -> (16.6163, 221.628) centre (0, 0) ccw projected
  arc A3 (14.7621, 233.2133) -> (9.6962, 233.4787) centre (0, 0) ccw projected
  arc A4 (6.6412, 222.1508) -> (1.1158, 222.2472) centre (0, 0) ccw projected
  arc A5 (-1.542, 233.6749) -> (-6.614, 233.5864) centre (0, 0) ccw projected
  arc A6 (-8.8715, 222.0729) -> (-14.3901, 221.7837) centre (0, 0) ccw projected
  arc A7 (-17.8386, 232.9981) -> (-22.8921, 232.556) centre (0, 0) ccw projected
  arc A8 (-24.3409, 220.9131) -> (-29.8259, 220.2396) centre (0, 0) ccw projected
  arc A9 (-34.0483, 231.1862) -> (-39.0586, 230.3926) centre (0, 0) ccw projected
  arc A10 (-39.6917, 218.677) -> (-45.1163, 217.6226) centre (0, 0) ccw projected
  arc A11 (-50.0921, 228.2479) -> (-55.0348, 227.1068) centre (0, 0) ccw projected
  arc A12 (-54.8491, 215.3756) -> (-60.187, 213.9453) centre (0, 0) ccw projected
  arc A13 (-65.8918, 224.1977) -> (-70.7429, 222.7146) centre (0, 0) ccw projected
  arc A14 (-69.7394, 211.0248) -> (-74.9645, 209.2257) centre (0, 0) ccw projected
  arc A15 (-81.3706, 219.0552) -> (-86.1064, 217.2373) centre (0, 0) ccw projected
  arc A16 (-84.2898, 205.646) -> (-89.3767, 203.4868) centre (0, 0) ccw projected
  arc A17 (-96.4529, 212.8454) -> (-101.0504, 210.7016) centre (0, 0) ccw projected
  arc A18 (-98.4297, 199.2653) -> (-103.3535, 196.7565) centre (0, 0) ccw projected
  arc A19 (-111.0653, 205.5988) -> (-115.502, 203.1394) centre (0, 0) ccw projected
  arc A20 (-112.0899, 191.9138) -> (-116.8268, 189.0676) centre (0, 0) ccw projected
  arc A21 (-125.1366, 197.3504) -> (-129.3909, 194.5876) centre (0, 0) ccw projected
  arc A22 (-125.2041, 183.6273) -> (-129.7309, 180.4576) centre (0, 0) ccw projected
  arc A23 (-138.5982, 188.1406) -> (-142.6495, 185.0877) centre (0, 0) ccw projected
  arc A24 (-137.7083, 174.4462) -> (-142.003, 170.9685) centre (0, 0) ccw projected
  arc A25 (-151.3846, 178.0142) -> (-155.2131, 174.6861) centre (0, 0) ccw projected
  arc A26 (-149.5416, 164.4152) -> (-153.5832, 160.6464) centre (0, 0) ccw projected
  arc A27 (-163.4335, 167.0205) -> (-167.0205, 163.4335) centre (0, 0) ccw projected
  arc A28 (-160.6464, 153.5832) -> (-164.4152, 149.5416) centre (0, 0) ccw projected
  arc A29 (-174.6861, 155.2131) -> (-178.0142, 151.3846) centre (0, 0) ccw projected
  arc A30 (-170.9685, 142.003) -> (-174.4462, 137.7083) centre (0, 0) ccw projected
  arc A31 (-185.0877, 142.6495) -> (-188.1406, 138.5982) centre (0, 0) ccw projected
  arc A32 (-180.4576, 129.7309) -> (-183.6273, 125.2041) centre (0, 0) ccw projected
  arc A33 (-194.5876, 129.3909) -> (-197.3504, 125.1366) centre (0, 0) ccw projected
  arc A34 (-189.0676, 116.8268) -> (-191.9138, 112.0899) centre (0, 0) ccw projected
  arc A35 (-203.1394, 115.502) -> (-205.5988, 111.0653) centre (0, 0) ccw projected
  arc A36 (-196.7565, 103.3535) -> (-199.2653, 98.4297) centre (0, 0) ccw projected
  arc A37 (-210.7016, 101.0504) -> (-212.8454, 96.4529) centre (0, 0) ccw projected
  arc A38 (-203.4868, 89.3767) -> (-205.646, 84.2898) centre (0, 0) ccw projected
  arc A39 (-217.2373, 86.1064) -> (-219.0552, 81.3706) centre (0, 0) ccw projected
  arc A40 (-209.2257, 74.9645) -> (-211.0248, 69.7394) centre (0, 0) ccw projected
  arc A41 (-222.7146, 70.7429) -> (-224.1977, 65.8918) centre (0, 0) ccw projected
  arc A42 (-213.9453, 60.187) -> (-215.3756, 54.8491) centre (0, 0) ccw projected
  arc A43 (-227.1068, 55.0348) -> (-228.2479, 50.0921) centre (0, 0) ccw projected
  line L0 (-228.2479, 50.0921) -> (-8.1092, -24.0707) projected
  arc A44 (-8.1092, -24.0707) -> (25.2107, -3.0955) centre (0, 0) ccw projected
  line L1 (25.2107, -3.0955) -> (49.9745, 198.5899) projected
  arc A45 (49.9745, 198.5899) -> (38.7871, 222.8634) centre (24.7639, 201.6854) ccw projected
  spline S0 degree 2 poles (38.7871, 222.8634) (38.113, 221.0698) (37.4939, 219.0645) knots 0 0 0 1 1 1 projected
  arc A46 (37.4939, 219.0645) -> (32.0358, 219.929) centre (0, 0) ccw projected
  circle A47 centre (0, 0) radius 14.2875 projected
  circle A48 centre (24.7639, 201.6854) radius 14.2875 projected
  arc A49 (49.2615, 208.3953) -> (37.4939, 219.0645) centre (34.9993, 204.4889) ccw
  arc A50 (49.9745, 198.5899) -> (38.7871, 222.8634) centre (24.7639, 201.6854) ccw projected
  constraints: 3 point on circle, 2 tangent, 1 centre point, 44 other
extrude "Extrusion13" cut sketch "Sketch12" against normal blind 6.35 contours A49 S0 A45
equation "\"PD\" = 457.2"
equation "\"a\" = 14.5deg"
equation "\"add\" = mod"
equation "\"ded\" = 6.35"
equation "\"RD\" = PD - 2 * ded"
equation "\"OD\" = PD + 2 * add"
equation "\"mod\" = 5.08"
body "Solid2"
